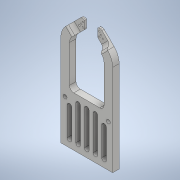
# Autodesk Inventor part: twoSidedHeadplateHolder_NP_v02
Saved by Autodesk Inventor 2022.1 (Build 261234000, 234)
## iProperties
Created: 2019-03-20
Part Number: twoSidedHeadplateHolder_NP_v02
Material: Generic
Document SubType Name: Modeling
Designer: Wilson Lab
Density: 1 g/cm^3
Appearance: Default
Author: Wilson Lab
Autodesk Inventor part; units mm, degrees
ref_plane "YZ Plane" through (0, 0, 0) normal (1, 0, 0) x (0, 1, 0)
ref_plane "XZ Plane" through (0, 0, 0) normal (0, 1, 0) x (-1, 0, 0)
ref_plane "XY Plane" through (0, 0, 0) normal (0, 0, 1) x (1, 0, 0)
sketch "Sketch1" plane through (0, 0, 0) normal (0, 0, 1) x (1, 0, 0)
  circle A0 centre (48.5717, 24.7756) radius 3.429
  circle A1 centre (54.9217, 50.1756) radius 2.794
  circle A2 centre (-2.2283, 24.7756) radius 3.429
  circle A3 centre (-8.5783, 50.1756) radius 2.794
  arc A4 (12.3675, 142.0509) -> (13.2975, 144.2959) centre (10.1225, 144.2959) ccw
  circle A5 centre (23.1717, 24.7756) radius 3.429
  arc A6 (13.7737, 50.1756) -> (7.1697, 50.1756) centre (10.4717, 50.1756) ccw
  line L0 (7.1697, 50.1756) -> (7.1697, -0.6244)
  line L1 (13.7737, 50.1756) -> (13.7737, -0.6244)
  line L2 (-14.9283, 61.3516) -> (-14.9283, -11.8004)
  arc A7 (7.1697, -0.6244) -> (13.7737, -0.6244) centre (10.4717, -0.6244) ccw
  line L3 (-14.9283, -11.8004) -> (23.1717, -11.8004)
  line L4 (32.5697, 50.1756) -> (32.5697, -0.6244)
  line L5 (39.1737, 50.1756) -> (39.1737, -0.6244)
  arc A8 (32.5697, -0.6244) -> (39.1737, -0.6244) centre (35.8717, -0.6244) ccw
  line L6 (61.2717, -11.8004) -> (23.1717, -11.8004)
  line L7 (61.2717, 61.3516) -> (61.2717, -11.8004)
  line L8 (42.2217, 61.3516) -> (23.1717, 61.3516)
  line L9 (4.1217, 61.3516) -> (23.1717, 61.3516)
  arc A9 (-2.2283, 67.7016) -> (4.1217, 61.3516) centre (4.1217, 67.7016) ccw
  arc A10 (39.1737, 50.1756) -> (32.5697, 50.1756) centre (35.8717, 50.1756) ccw
  circle A11 centre (40.3485, 144.9938) radius 1.1303
  circle A12 centre (37.5862, 148.3847) radius 1.1303
  circle A13 centre (35.2685, 144.9938) radius 1.1303
  circle A14 centre (35.2685, 151.7756) radius 1.1303
  arc A15 (42.2217, 61.3516) -> (48.5717, 67.7016) centre (42.2217, 67.7016) ccw
  line L10 (48.5717, 67.7016) -> (48.5717, 122.1945)
  line L11 (33.9759, 142.0509) -> (44.852, 131.1748)
  line L12 (33.046, 154.7283) -> (33.046, 144.2959)
  arc A16 (34.316, 155.9983) -> (33.046, 154.7283) centre (34.316, 154.7283) ccw
  circle A17 centre (5.995, 144.9938) radius 1.1303
  circle A18 centre (8.7572, 148.3847) radius 1.1303
  circle A19 centre (11.075, 144.9938) radius 1.1303
  circle A20 centre (11.075, 151.7756) radius 1.1303
  line L13 (61.2717, 61.3516) -> (61.2717, 122.3315)
  line L14 (-14.9283, 61.3516) -> (-14.9283, 122.3315)
  line L15 (12.3675, 142.0509) -> (1.4915, 131.1748)
  line L16 (12.0275, 155.9983) -> (9.5326, 155.9983)
  line L17 (7.2875, 155.0684) -> (-7.4888, 140.292)
  arc A21 (-7.4888, 140.292) -> (-14.9283, 122.3315) centre (10.4717, 122.3315) ccw
  arc A22 (61.2717, 122.3315) -> (53.8322, 140.292) centre (35.8717, 122.3315) ccw
  arc A23 (33.046, 144.2959) -> (33.9759, 142.0509) centre (36.221, 144.2959) ccw
  line L18 (39.0559, 155.0684) -> (53.8322, 140.292)
  line L19 (34.316, 155.9983) -> (36.8109, 155.9983)
  line L20 (-2.2283, 67.7016) -> (-2.2283, 122.1945)
  arc A24 (48.5717, 122.1945) -> (44.852, 131.1748) centre (35.8717, 122.1945) ccw
  arc A25 (13.2975, 154.7283) -> (12.0275, 155.9983) centre (12.0275, 154.7283) ccw
  arc A26 (1.4915, 131.1748) -> (-2.2283, 122.1945) centre (10.4717, 122.1945) ccw
  arc A27 (9.5326, 155.9983) -> (7.2875, 155.0684) centre (9.5326, 152.8233) ccw
  line L21 (13.2975, 154.7283) -> (13.2975, 144.2959)
  arc A28 (39.0559, 155.0684) -> (36.8109, 155.9983) centre (36.8109, 152.8233) ccw
  point P0 (0, 0)
  constraints: 44 end point, 32 point on circle, 29 centre point
extrude "Extrusion1" add sketch "Sketch1" along normal blind 9.525
sketch "Sketch2" plane through (0, 0, 9.525) normal (0, 0, 1) x (1, 0, 0)
  circle A0 centre (37.5862, 148.3847) radius 1.1303 projected
  circle A1 centre (8.7572, 148.3847) radius 1.1303 projected
  line L0 (37.5862, 148.3847) -> (8.7572, 148.3847) construction
  line L1 (23.1717, 148.3847) -> (23.1717, 160.1531) construction
  circle A2 centre (35.2685, 151.7756) radius 1.1303 projected
  line L2 (35.2685, 151.7756) -> (44.2487, 142.7953) construction
  line L3 (35.2685, 151.7756) -> (47.9685, 151.7756) construction
  line L4 (44.2487, 142.7953) -> (49.8381, 148.3847)
  line L5 (49.8381, 148.3847) -> (33.4899, 132.0365)
  line L6 (-3.4946, 148.3847) -> (12.8536, 132.0365)
  line L7 (12.8536, 132.0365) -> (33.4899, 132.0365)
  line L8 (49.8381, 148.3847) -> (33.4899, 164.7329)
  line L9 (-3.4946, 148.3847) -> (12.8536, 164.7329)
  line L10 (12.8536, 164.7329) -> (33.4899, 164.7329)
  point P0 (0, 0)
  point P1 (50.9684, 149.515)
  point P2 (-4.6249, 149.515)
  point P3 (50.9684, 147.2544)
  point P4 (-4.6249, 147.2544)
  dimension "d2" = 12.7
  dimension "d3" = 45
  constraints: 22 end point, 6 symmetric about line, 3 horizontal, 1 equal length, 1 midpoint, 1 perpendicular, 1 point on line, 1 vertical
  measures "d2" distance of L2.start L2.end
  measures "d3" angle of L2 L3
extrude "Extrusion2" cut sketch "Sketch2" against normal blind 6.35
fillet "Fillet1" radius 6.35 2 edges at (43.2645, 141.8111, 9.525) (3.079, 141.8111, 9.525) inverted yes
fillet "Fillet2" radius 3.175 1 edges at (47.7546, 137.3209, 9.525)
fillet "Fillet3" radius 3.175 1 edges at (-1.4112, 137.3209, 9.525)
sketch "Sketch3" plane through (0, 0, 9.525) normal (0, 0, 1) x (1, 0, 0)
  circle A0 centre (-2.2283, 24.7756) radius 3.429 construction
  circle A1 centre (23.1717, 24.7756) radius 3.429 construction
  arc A2 (-5.6573, -0.6244) -> (1.2007, -0.6244) centre (-2.2283, -0.6244) ccw
  line L0 (-5.6573, -0.6244) -> (-5.6573, 24.7756)
  line L1 (1.2007, -0.6244) -> (1.2007, 24.7756)
  arc A3 (19.7427, -0.6244) -> (26.6007, -0.6244) centre (23.1717, -0.6244) ccw
  line L2 (19.7427, -0.6244) -> (19.7427, 24.7756)
  line L3 (26.6007, -0.6244) -> (26.6007, 24.7756)
  arc A4 (45.1427, -0.6244) -> (52.0007, -0.6244) centre (48.5717, -0.6244) ccw
  line L4 (45.1427, -0.6244) -> (45.1427, 24.7756)
  line L5 (52.0007, -0.6244) -> (52.0007, 24.7756)
  arc A5 (1.2007, 41.275) -> (-5.6573, 41.275) centre (-2.2283, 41.275) ccw
  line L6 (-5.6573, 24.7756) -> (-5.6573, 41.275)
  line L7 (1.2007, 24.7756) -> (1.2007, 41.275)
  arc A6 (52.0007, 41.275) -> (45.1427, 41.275) centre (48.5717, 41.275) ccw
  line L8 (45.1427, 24.7756) -> (45.1427, 41.275)
  line L9 (52.0007, 24.7756) -> (52.0007, 41.275)
  arc A7 (26.6007, 50.1756) -> (19.7427, 50.1756) centre (23.1717, 50.1756) ccw
  line L10 (19.7427, 50.1756) -> (19.7427, 24.7756)
  line L11 (26.6007, 50.1756) -> (26.6007, 24.7756)
  point P0 (0, 0)
  constraints: 24 end point, 14 point on circle, 6 centre point, 5 tangent, 3 vertical, 2 equal length, 2 point on line
extrude "Extrusion3" cut sketch "Sketch3" against normal blind 25.4
body "Solid1"
